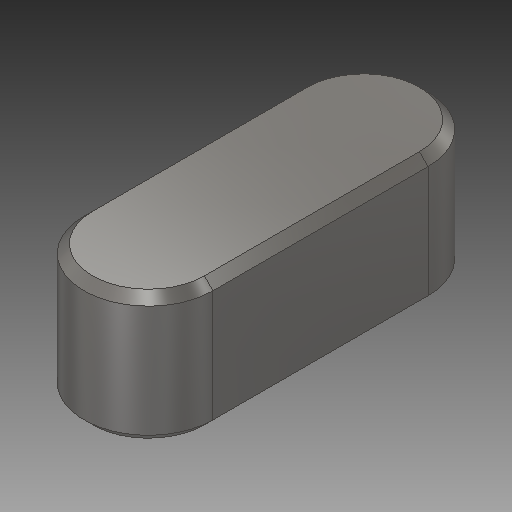
# Autodesk Inventor part: feather_key
Saved by Autodesk Inventor 2019.2 (Build 232265000, 265)
## iProperties
Created: 2018-11-26
Part Number: feather_key
Material: Stainless Steel
Document SubType Name: Modeling
Designer: Petar
Density: 8 g/cm^3
Appearance: Semi-Polished
d1: 5,000 mm
d2: 3,000 mm
d3: 0,00 deg
d4: 0,200 mm
d7: 3,000 mm
Author: Petar
Autodesk Inventor part; units mm, degrees
ref_plane "YZ Plane" through (0, 0, 0) normal (1, 0, 0) x (0, 1, 0)
ref_plane "XZ Plane" through (0, 0, 0) normal (0, 1, 0) x (-1, 0, 0)
ref_plane "XY Plane" through (0, 0, 0) normal (0, 0, 1) x (1, 0, 0)
sketch "Sketch1" plane through (0, 0, 0) normal (0, 1, 0) x (-1, 0, 0)
  line L0 (0.3129, 0) -> (0.3129, 5)
  line L1 (3.3129, 5) -> (3.3129, 0)
  arc A0 (3.3129, 5) -> (0.3129, 5) centre (1.8129, 5) ccw
  arc A1 (0.3129, 0) -> (3.3129, 0) centre (1.8129, 0) ccw
  point P0 (0, 0)
  dimension "d1" = 5
  dimension "d7" = 3
  constraints: 4 end point, 4 point on circle, 2 centre point, 1 parallel
  measures "d1" distance of L0.start L0.end
  measures "d7" distance between parallel lines of L0 L1
extrude "Extrusion1" add sketch "Sketch1" along normal blind 3
chamfer "Chamfer1" distance 0.2 angle 45 8 edges at (-0.3129, 3, 2.5) (-1.8129, 3, -1.5) (-1.8129, 3, 6.5) (-3.3129, 3, 2.5) (-0.3129, 0, 2.5) (-1.8129, 0, 6.5) (-3.3129, 0, 2.5) (-1.8129, 0, -1.5)
body "Solid1"
